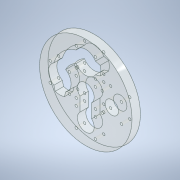
# Autodesk Inventor part: Middle_Plate_For_Valve
Saved by Autodesk Inventor 2020 (Build 240168000, 168)
## iProperties
Created: 2021-06-26
Part Number: Middle_Plate_For_Valve
Material: Glass
Document SubType Name: Modeling
Designer: Workshop
Density: 2.18 g/cm^3
Appearance: Clear
Author: Workshop
Autodesk Inventor part; units mm, degrees
ref_plane "YZ Plane" through (0, 0, 0) normal (1, 0, 0) x (0, 1, 0)
ref_plane "XZ Plane" through (0, 0, 0) normal (0, 1, 0) x (-1, 0, 0)
ref_plane "XY Plane" through (0, 0, 0) normal (0, 0, 1) x (1, 0, 0)
sketch "Sketch1" plane through (0, 0, 0) normal (0, 0, 1) x (1, 0, 0)
  line L0 (-6.9021, -7.2361) -> (-6.9021, -23.7397) projected
  arc A0 (-6.9021, -23.7397) -> (6.9021, -23.7397) centre (0, -30.9758) ccw projected
  line L1 (6.9021, -23.7397) -> (6.9021, -7.2361) projected
  arc A1 (6.9021, -7.2361) -> (-6.9021, -7.2361) centre (0, 0) ccw projected
  circle A2 centre (11.4021, -19.5736) radius 1.5 projected
  arc A3 (11.5492, 37.9661) -> (-11.5492, 37.9661) centre (0, 30.9758) ccw projected
  arc A4 (-11.5492, 37.9661) -> (-37.9661, 11.5492) centre (0, 0) ccw projected
  arc A5 (-37.9661, 11.5492) -> (-37.9661, -11.5492) centre (-30.9758, 0) ccw projected
  line L2 (-37.9661, -11.5492) -> (-36.4373, -17.1387) projected
  arc A6 (-36.4373, -17.1387) -> (-25.5143, -17.1387) centre (-30.9758, 0) ccw projected
  line L3 (-25.5143, -17.1387) -> (-23.9854, -11.5492) projected
  arc A7 (-23.9854, -11.5492) -> (-23.9854, 11.5492) centre (-30.9758, 0) ccw projected
  arc A8 (-11.5492, 23.9854) -> (-23.9854, 11.5492) centre (0, 0) ccw projected
  arc A9 (-11.5492, 23.9854) -> (11.5492, 23.9854) centre (0, 30.9758) ccw projected
  line L4 (11.5492, 23.9854) -> (17.1387, 25.5143) projected
  arc A10 (17.1387, 25.5143) -> (17.1387, 36.4373) centre (0, 30.9758) ccw projected
  line L5 (17.1387, 36.4373) -> (11.5492, 37.9661) projected
  circle A11 centre (-11.4021, 42.3778) radius 1.5 projected
  circle A12 centre (11.4021, -42.3778) radius 1.5 projected
  circle A13 centre (0, 0) radius 55 projected
  circle A14 centre (-11.4021, -11.4021) radius 1.5 projected
  circle A15 centre (-11.4021, 19.5736) radius 1.5 projected
  circle A16 centre (-19.5737, 11.4021) radius 1.5 projected
  circle A17 centre (-19.5736, -11.4021) radius 1.5 projected
  circle A18 centre (-42.3779, 11.4021) radius 1.5 projected
  circle A19 centre (-42.3778, -11.4021) radius 1.5 projected
  circle A20 centre (-11.4021, 11.4021) radius 1.5 projected
  circle A21 centre (11.4021, 11.4021) radius 1.5 projected
  circle A22 centre (11.4021, -11.4021) radius 1.5 projected
  circle A23 centre (11.4021, 19.5737) radius 1.5 projected
  circle A24 centre (19.5736, 11.4021) radius 1.5 projected
  circle A25 centre (19.5737, -11.4021) radius 1.5 projected
  circle A26 centre (11.4021, 42.3779) radius 1.5 projected
  circle A27 centre (30.9758, 0) radius 8 projected
  circle A28 centre (42.3779, -11.4021) radius 1.5 projected
  circle A29 centre (42.3778, 11.4021) radius 1.5 projected
  circle A30 centre (-11.4021, -19.5737) radius 1.5 projected
  circle A31 centre (-11.4021, -42.3779) radius 1.5 projected
extrude "Extrusion1" add sketch "Sketch1" along normal mid plane 10
body "Solid1"
